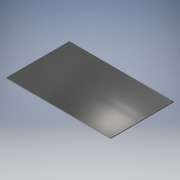
# Autodesk Inventor part: Cover_LiftSurface
Saved by Autodesk Inventor 2018 (Build 220112000, 112)
## iProperties
Created: 2017-11-14
Part Number: Cover_LiftSurface
Material: Steel, Galvanized
Document SubType Name: Modeling
Designer: P136265
Density: 7.85 g/cm^3
Appearance: Galvanized
Author: P136265
Autodesk Inventor part; units mm, degrees
ref_plane "YZ Plane" through (0, 0, 0) normal (1, 0, 0) x (0, 1, 0)
ref_plane "XZ Plane" through (0, 0, 0) normal (0, 1, 0) x (-1, 0, 0)
ref_plane "XY Plane" through (0, 0, 0) normal (0, 0, 1) x (1, 0, 0)
sketch "Sketch1" plane through (0, 0, 0) normal (0, 0, 1) x (1, 0, 0)
  line L0 (379.3, -228.3507) -> (379.3, 230.2493) construction
  line L1 (-379.3, 230.2493) -> (-379.3, -228.3507) construction
  line L2 (379.3, 230.2493) -> (-379.3, 230.2493) construction
  line L3 (379.3, -228.3507) -> (-379.3, -228.3507) construction
  line L4 (377.3, 230.2493) -> (-377.3, 230.2493)
  line L5 (-379.3, 228.2493) -> (-379.3, -226.3507)
  line L6 (-377.3, -228.3507) -> (377.3, -228.3507)
  line L7 (379.3, -226.3507) -> (379.3, 228.2493)
  arc A0 (377.3, -228.3507) -> (379.3, -226.3507) centre (377.3, -226.3507) ccw
  arc A1 (379.3, 228.2493) -> (377.3, 230.2493) centre (377.3, 228.2493) ccw
  arc A2 (-377.3, 230.2493) -> (-379.3, 228.2493) centre (-377.3, 228.2493) ccw
  arc A3 (-379.3, -226.3507) -> (-377.3, -228.3507) centre (-377.3, -226.3507) ccw
  point P0 (0, 0)
  dimension "d0" = 2
  constraints: 8 end point, 8 point on circle, 8 tangent, 4 centre point, 4 point on line, 3 equal radius, 2 parallel, 1 horizontal, 1 perpendicular
  measures "d0" radius of A0
extrude "Extrusion1" add sketch "Sketch1" along normal mid plane 5
body "Solid1"
